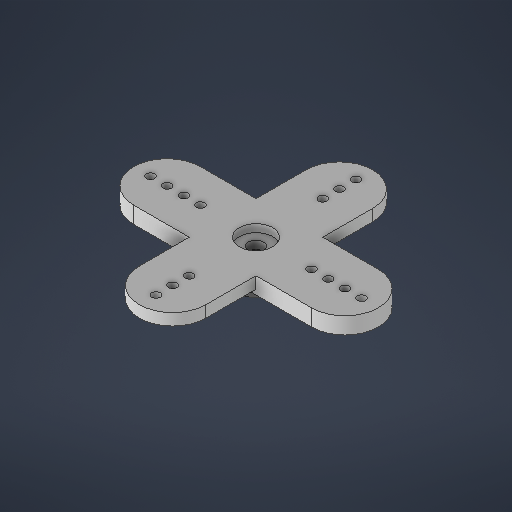
# Autodesk Inventor part: MMAE 232 CAD Assignment 2 Servo Horn 3-Nicholas Skiba
Saved by Autodesk Inventor 2026.1 (Build 301233000, 233)
## iProperties
Created: 2025-08-27
Part Number: MMAE 232 CAD Assignment 2 Servo Horn 3-Nicholas Skiba
Material: Generic
Document SubType Name: Modeling
Designer: Nick
Density: 1 g/cm^3
Appearance: Default
Author: Nick
Autodesk Inventor part; units mm, degrees
ref_plane "YZ Plane" through (0, 0, 0) normal (1, 0, 0) x (0, 1, 0)
ref_plane "XZ Plane" through (0, 0, 0) normal (0, 1, 0) x (-1, 0, 0)
ref_plane "XY Plane" through (0, 0, 0) normal (0, 0, 1) x (1, 0, 0)
sketch "Sketch1" plane through (0, 0, 0) normal (0, 1, 0) x (-1, 0, 0)
  line L0 (0, 0) -> (0, -15) construction
  line L1 (0, 0) -> (16, 0) construction
  arc A0 (-6, -15) -> (6, -15) centre (0, -15) ccw
  arc A1 (16, -6) -> (16, 6) centre (16, 0) ccw
  line L2 (-6, -15) -> (-6, -6)
  line L3 (0, -6) -> (-6, -6) construction
  line L4 (16, 6) -> (6, 6)
  line L5 (6, 6) -> (-6, 6) construction
  line L6 (-6, 6) -> (-6, -6) construction
  line L7 (16, -6) -> (6, -6)
  line L8 (6, -6) -> (0, -6) construction
  line L9 (6, -15) -> (6, -6)
  circle A2 centre (0, 0) radius 1.35
  line L10 (0, 0) -> (0, -12) construction
  line L11 (0, -12) -> (0, -15) construction
  line L12 (0, -15) -> (0, -18) construction
  line L13 (0, 0) -> (10, 0) construction
  line L14 (10, 0) -> (13, 0) construction
  line L15 (13, 0) -> (16, 0) construction
  line L16 (16, 0) -> (19, 0) construction
  circle A3 centre (19, 0) radius 0.75
  circle A4 centre (16, 0) radius 0.75
  circle A5 centre (13, 0) radius 0.75
  circle A6 centre (10, 0) radius 0.75
  circle A7 centre (0, -12) radius 0.75
  circle A8 centre (0, -15) radius 0.75
  circle A9 centre (0, -18) radius 0.75
  line L17 (6.8305, 0) -> (-5.2, 0)
  line L18 (0, -4.7373) -> (0, 4.2525)
  arc A10 (6, 15) -> (-6, 15) centre (0, 15) ccw
  line L19 (-6, 15) -> (-6, 6)
  line L20 (6, 15) -> (6, 6)
  circle A11 centre (0, 12) radius 0.75
  circle A12 centre (0, 15) radius 0.75
  circle A13 centre (0, 18) radius 0.75
  arc A14 (-16, 6) -> (-16, -6) centre (-16, 0) ccw
  line L21 (-16, 6) -> (-6, 6)
  line L22 (-16, -6) -> (-6, -6)
  circle A15 centre (-19, 0) radius 0.75
  circle A16 centre (-16, 0) radius 0.75
  circle A17 centre (-13, 0) radius 0.75
  circle A18 centre (-10, 0) radius 0.75
  dimension "d0" = 15
  dimension "d1" = 16
  dimension "d2" = 12
  dimension "d3" = 12
  dimension "d5" = 2.7
  dimension "d6" = 12
  dimension "d7" = 3
  dimension "d8" = 3
  dimension "d9" = 10
  dimension "d10" = 3
  dimension "d11" = 3
  dimension "d12" = 3
  dimension "d13" = 1.5
  dimension "d14" = 1.5
  dimension "d15" = 1.5
  dimension "d16" = 1.5
  dimension "d17" = 1.5
  dimension "d18" = 1.5
  dimension "d19" = 1.5
  dimension "d20" = 6
  constraints: 46 end point, 19 centre point, 13 symmetric about line, 11 coincident, 11 point on line, 8 point on circle, 4 perpendicular, 3 collinear, 3 horizontal, 3 tangent, 2 vertical, 9 other
  measures "d0" distance of L0.start L0.end
  measures "d1" distance of L0.start L1.end
  measures "d2" diameter of A0
  measures "d3" diameter of A1
  measures "d5" diameter of A2
  measures "d6" distance of L10.start L10.end
  measures "d7" distance of L10.end L11.end
  measures "d8" distance of L11.end L12.end
  measures "d9" distance of L10.start L13.end
  measures "d10" distance of L13.end L14.end
  measures "d11" distance of L14.end L15.end
  measures "d12" distance of L15.end L16.end
  measures "d13" diameter of A3
  measures "d14" diameter of A4
  measures "d15" diameter of A5
  measures "d16" diameter of A6
  measures "d17" diameter of A7
  measures "d18" diameter of A8
  measures "d19" diameter of A9
  measures "d20" distance from line of L0.start L20
extrude "Extrusion1" add sketch "Sketch1" along normal blind 2.1
sketch "Sketch2" plane through (0, 2.1, 0) normal (0, 1, 0) x (1, 0, 0)
  circle A0 centre (0, 0) radius 3
  dimension "d23" = 6
  constraints: 1 centre point, 1 coincident
  measures "d23" diameter of A0
extrude "Extrusion2" cut sketch "Sketch2" against normal blind 1.4
sketch "Sketch3" plane through (0, 0, 0) normal (0, -1, 0) x (1, 0, 0)
  circle A0 centre (0, 0) radius 1.35 projected
  circle A1 centre (0, 0) radius 6
  dimension "d26" = 12
  constraints: 1 centre point, 1 coincident
  measures "d26" diameter of A1
extrude "Extrusion3" add sketch "Sketch3" along normal blind 0.9
sketch "Sketch4" plane through (0, -0.9, 0) normal (0, -1, 0) x (1, 0, 0)
  circle A0 centre (0, 0) radius 1.35 projected
  circle A1 centre (0, 0) radius 5
  dimension "d29" = 10
  constraints: 1 centre point, 1 coincident
  measures "d29" diameter of A1
extrude "Extrusion4" add sketch "Sketch4" along normal blind 2.85
sketch "Sketch5" plane through (0, 0, 0) normal (0, -1, 0) x (1, 0, 0)
  line L0 (16, -6) -> (6, -6) projected
  arc A0 (-16, 6) -> (-16, -6) centre (-16, 0) ccw projected
  line L1 (16, -6) -> (-16, -6)
  line L2 (6, 6) -> (16, 6) projected
  line L3 (16, 6) -> (-16, 6)
  circle A1 centre (-16, 0) radius 0.75 projected
  arc A2 (-16, 6) -> (-16, -6) centre (-16, 0) ccw
  circle A3 centre (16, 0) radius 0.75 projected
  arc A4 (16, -6) -> (16, 6) centre (16, 0) ccw
  circle A5 centre (-10, 0) radius 0.75 projected
  circle A6 centre (-10, 0) radius 0.75
  circle A7 centre (-13, 0) radius 0.75 projected
  circle A8 centre (-13, 0) radius 0.75
  circle A9 centre (-19, 0) radius 0.75 projected
  circle A10 centre (-19, 0) radius 0.75
  circle A11 centre (-16, 0) radius 0.75
  circle A12 centre (10, 0) radius 0.75 projected
  circle A13 centre (10, 0) radius 0.75
  circle A14 centre (13, 0) radius 0.75 projected
  circle A15 centre (13, 0) radius 0.75
  circle A16 centre (16, 0) radius 0.75
  circle A17 centre (19, 0) radius 0.75 projected
  circle A18 centre (19, 0) radius 0.75
  point P0 (0, 0)
  constraints: 10 centre point, 10 coincident, 4 end point, 4 point on circle, 2 concentric, 1 collinear, 1 horizontal, 1 tangent
extrude "Extrusion5" add sketch "Sketch5" along normal blind 0.9
sketch "Sketch6" plane through (0, -0.9, 0) normal (0, -1, 0) x (1, 0, 0)
  circle A0 centre (0, 0) radius 1.35 projected
  circle A1 centre (0, 0) radius 1.35
  constraints: 1 centre point, 1 coincident
extrude "Extrusion6" cut sketch "Sketch6" against normal blind 0.9
sketch "Sketch7" plane through (0, -3.75, 0) normal (0, -1, 0) x (1, 0, 0)
  circle A0 centre (0, 0) radius 1.35 projected
  circle A1 centre (0, 0) radius 2.75
  dimension "d36" = 5.5
  constraints: 1 centre point, 1 coincident
  measures "d36" diameter of A1
extrude "Extrusion7" cut sketch "Sketch7" against normal blind 3 contours A0 | A1
body "Solid1"
